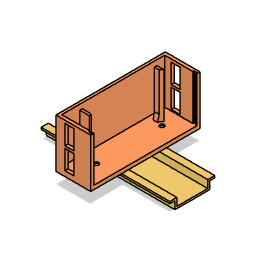
WLEDBoardMount (Autodesk Fusion 360 design; units mm, degrees)
Autodesk Fusion 360 part; units mm, degrees
sketch "Skizze1" plane through (0, 0, 0) normal (1, 0, 0) x (0, 0, -1) in component "Rail"
  line L0 (-17.5, 0) -> (17.5, 0)
  line L1 (-12, 0) -> (-12, -6)
  line L2 (-12, -6) -> (12, -6)
  line L3 (13.5, -1.5) -> (17.5, -1.5)
  line L4 (17.5, 0) -> (17.5, -1.5)
  line L5 (12, -6) -> (12, 0)
  line L6 (13.5, -7.5) -> (13.5, -1.5)
  line L7 (0, -7.5) -> (0, 0) construction
  line L8 (-17.5, 0) -> (-17.5, -1.5)
  line L9 (-17.5, -1.5) -> (-13.5, -1.5)
  line L10 (-13.5, -1.5) -> (-13.5, -7.5)
  line L11 (-13.5, -7.5) -> (13.5, -7.5)
  point P0 (0, -26.5)
  point P1 (5, -20.5)
  point P2 (5, -17.5)
  point P3 (-5, -17.5)
  point P4 (5, -20.5)
  point P5 (5, -17.5)
  point P6 (0, -26.5)
  point P7 (0, -8.5)
  point P8 (0, -14.5)
  point P9 (0, -35.0071)
  point P10 (0, -2.5)
  point P11 (0, 3.5)
  point P12 (0, 27.7571)
  point P13 (0, -0.2)
  point P14 (0, -8.5)
  point P15 (0, -14.5)
  point P16 (0, -35.0071)
  point P17 (0, -2.5)
  point P18 (0, 3.5)
  point P19 (0, 27.7571)
  point P20 (0, -0.2)
  point P21 (0, 24.5)
  point P22 (0, 24.5)
  point P23 (-50, 12)
  point P24 (50, 12)
  point P25 (50, 17.5)
  point P26 (-50, 17.5)
  point P27 (0, -24.5)
  point P28 (0, 26.5)
  point P29 (0, -26.5)
  point P30 (0, 24.5)
  point P31 (-7.5, 4)
  point P32 (-7.5, 39)
  dimension "d58" = 1
  dimension "d59" = 5
  constraint horizontal L0
  constraint midpoint L7.end L0
  constraint horizontal L11
  constraint midpoint L7.start L11
  constraint coincident L7.end origin
  constraint vertical L7
  constraint perpendicular L0 L8
  constraint perpendicular L0 L4
  constraint perpendicular L6 L11
  constraint perpendicular L3 L4
  constraint perpendicular L6 L9
  constraint perpendicular L9 L10
  constraint equal L4 L8
  constraint coincident L1.start L0
  constraint perpendicular L0 L1
  constraint perpendicular L2 L6
  constraint coincident L5.end L0
  constraint perpendicular L0 L5
  measures "d1" distance of L0.start L0.end
  measures "d2" distance of L10.end L6.start
  measures "d3" distance of L3.end L0.end
  measures "d4" distance of L0 L11
  measures "d5" distance of L2 L11
  measures "d6" distance of L1 L10
  measures "d7" distance of L5 L6
extrude "Extrusion1" add sketch "Skizze1" along normal mid plane 100 contours L0 L1 L2 L3 L4 L5 L6 L8 L9 L10 L11 makes body 1 in component "Rail"
sketch "Skizze1 (2)" plane through (0, 0, 0) normal (0, 1, 0) x (1, 0, 0) in component "DinRailMount"
  line L0 (-80, 17.5) -> (80, 17.5)
  line L1 (-80, 12) -> (80, 12)
  line L2 (-80, -12) -> (80, -12)
  line L3 (80, -17.5) -> (-80, -17.5)
  line L4 (0, 17.5) -> (0, -17.5) construction
  line L5 (-5, 17.5) -> (5, 17.5)
  line L6 (5, 17.5) -> (5, 20.5)
  line L7 (5, 20.5) -> (-5, 20.5)
  line L8 (-5, 20.5) -> (-5, 17.5)
  arc A0 (0, 17.5) -> (0, 11.5) centre (0, 14.5) ccw
  arc A1 (0, 5.5) -> (0, 11.5) centre (0, 8.5) ccw
  arc A2 (0, 5.5) -> (0, -0.5) centre (0, 2.5) ccw
  arc A3 (0, -6.5) -> (0, -0.5) centre (0, -3.5) ccw
  arc A4 (0, -5.8) -> (0, -1.2) centre (0, -3.5) ccw
  arc A5 (0, 6.2) -> (0, -1.2) centre (0, 2.5) ccw
  arc A6 (0, 6.2) -> (0, 10.8) centre (0, 8.5) ccw
  arc A7 (0, 18.2) -> (0, 10.8) centre (0, 14.5) ccw
  arc A8 (0, 16.8) -> (0, 12.2) centre (0, 14.5) ccw
  arc A9 (0, 4.8) -> (0, 12.2) centre (0, 8.5) ccw
  arc A10 (0, 4.8) -> (0, 0.2) centre (0, 2.5) ccw
  arc A11 (0, -7.2) -> (0, 0.2) centre (0, -3.5) ccw
  arc A12 (0, 16.8) -> (5, 17.5) centre (0, 35.0071) ccw
  line L9 (-8.5, 22.5) -> (8.5, 22.5) construction
  line L10 (8.5, 22.5) -> (8.5, -20.5)
  line L11 (8.5, -20.5) -> (-8.5, -20.5) construction
  line L12 (-8.5, -20.5) -> (-8.5, 22.5)
  line L13 (0, -17.5) -> (0, -20.5) construction
  line L14 (-5.5, 22.5) -> (5.5, 22.5)
  line L15 (5.5, 22.5) -> (5.5, -6.5)
  line L16 (5.5, -6.5) -> (-5.5, -6.5)
  line L17 (-5.5, -6.5) -> (-5.5, 22.5)
  arc A13 (0, -5.8) -> (-5.5, -6.5) centre (0, -27.7571) ccw
  line L18 (8.5, 22.5) -> (8.5, 30.5)
  line L19 (8.5, 30.5) -> (-8.5, 30.5)
  line L20 (-8.5, 30.5) -> (-8.5, 22.5)
  line L21 (0, 30.5) -> (0, 22.5) construction
  circle A14 centre (0, 26.5) radius 1.75
  line L22 (-8.5, -20.5) -> (-8.5, -28.5)
  line L23 (-8.5, -28.5) -> (8.5, -28.5)
  line L24 (8.5, -28.5) -> (8.5, -20.5)
  circle A15 centre (0, -24.5) radius 1.75
  line L25 (0, -28.5) -> (0, -20.5) construction
  line L26 (-50, 12) -> (50, 12)
  line L27 (50, 12) -> (50, 17.5)
  line L28 (50, 17.5) -> (-50, 17.5)
  line L29 (-50, 17.5) -> (-50, 12)
  dimension "d89_1" = 10
  dimension "d91_1" = 3
  dimension "d94_1" = 3
  dimension "d95_1" = 6
  dimension "d98_1" = 0
  dimension "d99_1" = -12
  dimension "d100_1" = 0.7
  dimension "d101_1" = -0.7
  dimension "d102_1" = 5
  dimension "d103_1" = 3
  dimension "d105_1" = 2
  dimension "d106_1" = 3.5
  dimension "d107_1" = 4
  dimension "d111_1" = 0.5
  dimension "d149_1" = 3
  constraint midpoint L0 L4.start
  constraint midpoint L3 L4.end
  constraint horizontal L5
  constraint vertical L6
  constraint horizontal L7
  constraint vertical L8
  constraint coincident L0 L5.start
  constraint midpoint L4.start L5
  constraint coincident L4 A0.end
  constraint coincident L4 A0.centre
  constraint coincident L4 A1.start
  constraint coincident L4 A1.centre
  constraint tangent A8 A12
  constraint horizontal L9
  constraint vertical L10
  constraint horizontal L11
  constraint vertical L12
  constraint midpoint L11 L13.end
  constraint collinear L4 L13
  constraint horizontal L14
  constraint vertical L15
  constraint horizontal L16
  constraint vertical L17
  constraint midpoint A3.start L16
  constraint tangent A4 A13
  constraint vertical L18
  constraint horizontal L19
  constraint vertical L20
  constraint coincident L9.end L10.start
  constraint midpoint L19 L21.start
  constraint midpoint L21 A14.centre
  constraint midpoint L14 L21.end
  constraint perpendicular L11 L22
  constraint perpendicular L22 L23
  constraint perpendicular L23 L24
  constraint equal L20 L22
  constraint equal A14 A15
  constraint midpoint L23 L25.start
  constraint midpoint A15.centre L25
  measures "d89_1" distance of L5.start L5.end
  measures "d91_1" distance of L5.end L6.end
  measures "d94_1" distance of L5 A0.centre
  measures "d95_1" distance of A0.centre A1.centre
  measures "d102_1" distance of L0 L9
  measures "d103_1" distance of L3 L11
  measures "d105_1" distance of L7 L14
  measures "d106_1" diameter of A14
  measures "d107_1" distance of L19 A14.centre
  measures "d111_1" distance of L8 L17
  measures "d149_1" distance of L12 L17
extrude "Extrusion1'" add sketch "Skizze1 (2)" along normal blind 3 separate body contours L0 L5 L6 L7 L8 L28 | L0 L1 L5 A0 A7 L26 L28 | L0 L1 L5 A0 A8 A9 A12 L26 L28 | L1 A0 A1 A2 A3 A4 A5 A6 A7 L16 A13 L26 | L1 A0 A1 A2 A3 A9 A10 A11 L16 L26 | L0 L10 L12 L14 L15 L17 L18 L19 L20 L28 | L0 L1 L10 L15 L26 L28 | L1 L2 L10 L12 L15 L16 L17 L26 | L0 L1 L12 L17 L26 L28 | L2 L3 L10 L12 | L3 L10 L12 L22 L23 L24 makes body 2 in component "DinRailMount"
sketch "Skizze2" plane through (0, 3, 0) normal (0, 1, 0) x (-1, 0, 0) in component "DinRailMount"
  circle A0 centre (0, -26.5) radius 1.75
  line L0 (5.5, 6.5) -> (5.5, -22.5)
  line L1 (5.5, -22.5) -> (-5.5, -22.5)
  line L2 (-5.5, -22.5) -> (-5.5, 6.5)
  line L3 (-5.5, 6.5) -> (-2.1656, 6.5)
  line L4 (-8.5, 28.5) -> (-8.5, -30.5)
  line L5 (-8.5, -30.5) -> (8.5, -30.5)
  line L6 (8.5, -30.5) -> (8.5, 28.5)
  line L7 (5, -17.5) -> (6, -17.5)
  line L8 (6, -17.5) -> (6, -22)
  line L9 (6, -22) -> (5.5, -22)
  line L10 (5, -20.5) -> (6, -20.5)
  line L11 (5, -17) -> (6.5, -17)
  line L12 (6.5, -17) -> (6.5, -22.5)
  line L13 (6.5, -22.5) -> (5.5, -22.5)
  line L14 (-5, -17.5) -> (-6, -17.5)
  line L15 (-6, -17.5) -> (-6, -22)
  line L16 (-6, -22) -> (-5.5, -22)
  line L17 (-5, -20.5) -> (-6, -20.5)
  line L18 (-5, -17) -> (-6.5, -17)
  line L19 (-6.5, -17) -> (-6.5, -22.5)
  line L20 (-6.5, -22.5) -> (-5.5, -22.5)
  line L21 (5, -20.5) -> (5, -17.5)
  line L22 (5, -17.5) -> (2.1656, -17.5)
  line L23 (-5, -17.5) -> (-5, -20.5)
  line L24 (-5, -20.5) -> (5, -20.5)
  line L25 (-5, -17.5) -> (-5, -20.5)
  line L26 (-5, -20.5) -> (5, -20.5)
  line L27 (5, -20.5) -> (5, -17.5)
  line L28 (5, -17.5) -> (2.1656, -17.5)
  line L29 (-8.5, 28.5) -> (-8.5, -30.5)
  line L30 (-8.5, -30.5) -> (8.5, -30.5)
  line L31 (8.5, -30.5) -> (8.5, 28.5)
  circle A1 centre (0, -26.5) radius 1.75
  line L32 (5.5, 6.5) -> (5.5, -22.5)
  line L33 (5.5, -22.5) -> (-5.5, -22.5)
  line L34 (-5.5, -22.5) -> (-5.5, 6.5)
  line L35 (-5.5, 6.5) -> (-2.1656, 6.5)
  arc A2 (0, -4.8) -> (0, -12.2) centre (0, -8.5) ccw
  arc A3 (0, -16.8) -> (0, -12.2) centre (0, -14.5) ccw
  arc A4 (0, -16.8) -> (-5, -17.5) centre (0, -35.0071) ccw
  arc A5 (2.1656, -17.5) -> (0, -10.8) centre (0, -14.5) ccw
  arc A6 (0, -6.2) -> (0, -10.8) centre (0, -8.5) ccw
  arc A7 (0, -6.2) -> (0, 1.2) centre (0, -2.5) ccw
  arc A8 (0, 5.8) -> (0, 1.2) centre (0, 3.5) ccw
  arc A9 (0, 5.8) -> (5.5, 6.5) centre (0, 27.7571) ccw
  arc A10 (-2.1656, 6.5) -> (0, -0.2) centre (0, 3.5) ccw
  arc A11 (0, -4.8) -> (0, -0.2) centre (0, -2.5) ccw
  arc A12 (0, -4.8) -> (0, -12.2) centre (0, -8.5) ccw
  arc A13 (0, -16.8) -> (0, -12.2) centre (0, -14.5) ccw
  arc A14 (0, -16.8) -> (-5, -17.5) centre (0, -35.0071) ccw
  arc A15 (2.1656, -17.5) -> (0, -10.8) centre (0, -14.5) ccw
  arc A16 (0, -6.2) -> (0, -10.8) centre (0, -8.5) ccw
  arc A17 (0, -6.2) -> (0, 1.2) centre (0, -2.5) ccw
  arc A18 (0, 5.8) -> (0, 1.2) centre (0, 3.5) ccw
  arc A19 (0, 5.8) -> (5.5, 6.5) centre (0, 27.7571) ccw
  arc A20 (-2.1656, 6.5) -> (0, -0.2) centre (0, 3.5) ccw
  arc A21 (0, -4.8) -> (0, -0.2) centre (0, -2.5) ccw
  line L36 (8.5, 28.5) -> (-8.5, 28.5)
  line L37 (8.5, 28.5) -> (-8.5, 28.5)
  circle A22 centre (0, 24.5) radius 1.75
  circle A23 centre (0, 24.5) radius 1.75
  dimension "d119_1" = 0.5
  dimension "d120_1" = -0.5
  dimension "d121_1" = 0.5
  dimension "d148_1" = 0.5
  constraint perpendicular L1 L8
  constraint perpendicular L0 L9
  constraint coincident L8 L10.end
  constraint perpendicular L8 L10
  constraint coincident L0 L9.end
  constraint coincident L1 L0.end
  constraint perpendicular L2 L14
  constraint perpendicular L14 L15
  constraint coincident L2 L16.end
  constraint perpendicular L2 L16
  constraint coincident L15 L17.end
  constraint perpendicular L15 L17
  constraint equal L7 L14
  constraint equal L8 L15
  measures "d119_1" distance of L0 L8
  measures "d121_1" distance of L1 L9
extrude "Extrusion2" cut sketch "Skizze2" against normal blind 1.4 from surface at -0.5 contours L0 L7 L8 L9 L11 L12 L13 L32 | L0 L8 L9 L10 L32 | L0 L7 L8 L10 L32 | L2 L14 L15 L16 L18 L19 L20 L34 | L2 L15 L16 L17 L34 | L2 L14 L15 L17 L34 bodies 2 in component "DinRailMount"
extrude "Extrusion3" add sketch "Skizze2" along normal blind 1 from surface at -1.7 contours L0 L7 L10 L21 L27 L32 | L0 L7 L8 L10 L32 | L2 L14 L17 L23 L25 L34 | L2 L14 L15 L17 L34 bodies 2 in component "DinRailMount"
sketch "Skizze3" plane through (5, 0, 0) normal (1, 0, 0) x (0, 0, -1) in component "DinRailMount"
  line L0 (20.5, 1.3) -> (17.5, 1.3)
  line L1 (17.5, 0) -> (20.5, 0)
  line L2 (20.5, 0) -> (20.5, 1.3)
  line L3 (20.5, 0) -> (20.5, -2)
  line L4 (16, -2) -> (16, -1.5)
  line L5 (16, -2) -> (17, -3)
  line L6 (17, -3) -> (19.5, -3)
  line L7 (19.5, -3) -> (20.5, -2)
  line L8 (20.5, -2) -> (16, -2) construction
  line L9 (17.5, 1.3) -> (17.5, 0)
  line L10 (-17.5, 0) -> (-17.5, -1.5)
  line L11 (-17.5, -1.5) -> (-13.5, -1.5)
  line L12 (-13.5, -1.5) -> (-13.5, -7.5)
  line L13 (-13.5, -7.5) -> (13.5, -7.5)
  line L14 (13.5, -7.5) -> (13.5, -1.5)
  line L15 (13.5, -1.5) -> (17.5, -1.5)
  line L16 (17.5, -1.5) -> (17.5, 0)
  line L17 (17.5, 0) -> (12, 0)
  line L18 (12, 0) -> (12, -6)
  line L19 (12, -6) -> (-12, -6)
  line L20 (-12, -6) -> (-12, 0)
  line L21 (-12, 0) -> (-17.5, 0)
  dimension "d127_1" = 1.5
  dimension "d129_1" = 0.5
  dimension "d130_1" = 1.5
  dimension "d151_1" = 45
  dimension "d152_1" = 45
  constraint coincident L1.end L2.start
  constraint perpendicular L1 L3
  constraint coincident L4.end L15
  constraint perpendicular L4 L15
  constraint horizontal L6
  constraint perpendicular L4 L8
  measures "d127_1" distance of L4 L16
  measures "d129_1" distance of L4.start L4.end
  measures "d130_1" distance of L6 L15
  measures "d151_1" angle of L5 L8
  measures "d152_1" angle of L7 L8
extrude "Extrusion4" add sketch "Skizze3" against normal up to surface (10 mm away) contours L1 L3 L4 L5 L6 L7 L15 L16 bodies 2 in component "DinRailMount"
sketch "Skizze4" plane through (8.5, 0, 0) normal (1, 0, 0) x (0, 0, -1) in component "DinRailMount"
  line L0 (-28.5, 0) -> (30.5, 0)
  line L1 (30.5, 0) -> (30.5, 3)
  line L2 (30.5, 3) -> (-28.5, 3)
  line L3 (-20, -3) -> (-21, -2)
  line L4 (-17, -3) -> (-20, -3)
  line L5 (-16, -2) -> (-17, -3)
  line L6 (-16, -2) -> (-16, -1.5)
  line L7 (-16, -2) -> (-21, -2) construction
  line L8 (-28.5, 3) -> (-28.5, 0)
  line L9 (-21, -2) -> (-21, 0)
  line L10 (-17.5, 0) -> (-17.5, -1.5)
  line L11 (-17.5, -1.5) -> (-13.5, -1.5)
  line L12 (-13.5, -1.5) -> (-13.5, -7.5)
  line L13 (-13.5, -7.5) -> (13.5, -7.5)
  line L14 (13.5, -7.5) -> (13.5, -1.5)
  line L15 (13.5, -1.5) -> (17.5, -1.5)
  line L16 (17.5, -1.5) -> (17.5, 0)
  line L17 (17.5, 0) -> (12, 0)
  line L18 (12, 0) -> (12, -6)
  line L19 (12, -6) -> (-12, -6)
  line L20 (-12, -6) -> (-12, 0)
  line L21 (-12, 0) -> (-17.5, 0)
  dimension "d141_1" = 0.5
  dimension "d143_1" = 1.5
  dimension "d144_1" = 1.5
  dimension "d153_1" = 45
  dimension "d154_1" = 45
  dimension "d238_1" = 5
  constraint coincident L6.end L11
  constraint perpendicular L6 L11
  constraint perpendicular L6 L7
  constraint coincident L0 L9.end
  constraint perpendicular L0 L9
  measures "d141_1" distance of L5.start L6.end
  measures "d143_1" distance of L4 L11
  measures "d144_1" distance of L6 L10
  measures "d153_1" angle of L3 L7
  measures "d154_1" angle of L5 L7
  measures "d238_1" distance of L6 L9
extrude "Extrusion5" add sketch "Skizze4" against normal up to surface (17 mm away) contours L0 L3 L4 L5 L6 L9 L10 L11 bodies 2 in component "DinRailMount"
ref_plane "Arbeitsebene1" through (0, 1, -1) normal (0, 1, 0) x (1, 0, 0) in component "DinRailMount"
sketch "Skizze1 (3)" plane through (0, 1, 0) normal (0, 1, 0) x (1, 0, 0) in component "MainBody"
  line L0 (-13.5, 42.5) -> (13.5, 42.5)
  line L1 (13.5, 42.5) -> (13.5, -42.5)
  line L2 (13.5, -42.5) -> (-13.5, -42.5)
  line L3 (-13.5, -42.5) -> (-13.5, 42.5)
  line L4 (-13.5, 42.5) -> (13.5, -42.5) construction
  line L5 (13.5, 42.5) -> (-13.5, -42.5) construction
  line L6 (8.5, -28.5) -> (8.5, 30.5)
  line L7 (-8.5, -28.5) -> (8.5, -28.5)
  circle A0 centre (0, -24.5) radius 1.75
  line L8 (-8.5, 30.5) -> (-8.5, -28.5)
  line L9 (8.5, 30.5) -> (-8.5, 30.5)
  circle A1 centre (0, 26.5) radius 1.75
  dimension "d10" = 27
  dimension "d11" = 85
  constraint horizontal L0
  constraint perpendicular L0 L1
  constraint parallel L0 L2
  constraint parallel L1 L3
  constraint coincident L4 origin
  constraint coincident L5 origin
  measures "d10" distance of L1.end L2.end
  measures "d11" distance of L0.end L1.end
extrude "Extrusion1''" add sketch "Skizze1 (3)" along normal blind 3 separate body contours L0 L1 L2 L3 | L6 L7 L8 L9 makes body 3 in component "MainBody"
extrude "Extrusion2'" cut sketch "Skizze1 (3)" along normal up to surface (2 mm away) contours L6 L7 L8 L9 bodies 3 in component "MainBody"
sketch "Skizze2 (2)" plane through (0, 4, 0) normal (0, 1, 0) x (-1, 0, 0) in component "MainBody"
  circle A0 centre (0, -26.5) radius 1.75
  circle A1 centre (0, 24.5) radius 1.75
  line L0 (13.5, 42.5) -> (-13.5, 42.5)
  line L1 (-13.5, 42.5) -> (-13.5, -42.5)
  line L2 (-13.5, -42.5) -> (13.5, -42.5)
  line L3 (13.5, -42.5) -> (13.5, 42.5)
  line L4 (-11.5, -40) -> (11.5, -40)
  line L5 (11.5, -40) -> (11.5, 40)
  line L6 (11.5, 40) -> (-11.5, 40)
  line L7 (-11.5, 40) -> (-11.5, -40) construction
  line L8 (-11.5, -40) -> (11.5, 40) construction
  line L9 (11.5, -40) -> (-11.5, 40) construction
  line L10 (7.5, -30) -> (7.5, -28)
  line L11 (1.9365, -30) -> (7.5, -30)
  line L12 (7.5, -28) -> (3.7081, -28)
  arc A2 (1.9365, -30) -> (3.7081, -28) centre (0, -26.5) ccw
  line L13 (7.5, 28) -> (1.9365, 28)
  line L14 (0, 28.5) -> (0, 30)
  line L15 (0, 30) -> (7.5, 30)
  line L16 (7.5, 30) -> (7.5, 28)
  line L17 (0, 24.5) -> (0, 28.5) construction
  arc A3 (1.9365, 28) -> (0, 28.5) centre (0, 24.5) ccw
  line L18 (-12.5, -41) -> (-10.5, -41)
  line L19 (-10.5, -41) -> (-10.5, -40)
  line L20 (-12.5, -41) -> (-12.5, -40)
  line L21 (-10.5, 40) -> (-10.5, 41)
  line L22 (-10.5, 41) -> (-12.5, 41)
  line L23 (-12.5, 41) -> (-12.5, 40)
  line L24 (-11.5, -40) -> (-13.5, -40)
  line L25 (-11.5, 40) -> (-13.5, 40)
  dimension "d18" = 2
  dimension "d19" = 80
  dimension "d31" = 8
  dimension "d32" = 2
  dimension "d33" = 10
  dimension "d35" = 10
  dimension "d62" = 1.5
  dimension "d64" = 2
  dimension "d65" = 1
  dimension "d66" = 4
  constraint horizontal L4
  constraint perpendicular L4 L5
  constraint parallel L4 L6
  constraint parallel L5 L7
  constraint coincident L8 origin
  constraint coincident L9 origin
  constraint vertical L10
  constraint horizontal L12
  constraint coincident A0.centre A2.centre
  constraint horizontal L11
  constraint horizontal L13
  constraint vertical L14
  constraint horizontal L15
  constraint vertical L16
  constraint concentric A1 A3
  constraint collinear L10 L16
  constraint equal L10 L16
  constraint coincident A1.centre L17.start
  constraint vertical L17
  constraint coincident L14.start L17.end
  constraint equal A2 A3
  constraint coincident L4 L20.end
  constraint perpendicular L4 L20
  constraint perpendicular L21 L22
  constraint coincident L6 L23.end
  constraint perpendicular L6 L23
  constraint collinear L19 L21
  constraint equal L18 L22
  constraint equal L20 L23
  constraint coincident L1 L24.end
  constraint perpendicular L1 L24
  constraint coincident L1 L25.end
  constraint perpendicular L1 L25
  constraint coincident L12.end A2.end
  constraint coincident L11.start A2.start
  constraint coincident L13.end A3.start
  constraint coincident L6 L21.start
  constraint coincident L4 L19.end
  measures "d18" distance of L1 L7
  measures "d19" distance of L4.start L6.end
  measures "d31" diameter of A2
  measures "d32" distance of L11 L12
  measures "d33" distance of L4 L11
  measures "d35" distance of L6 L15
  measures "d62" distance of L2 L18
  measures "d64" distance of L18.start L18.end
  measures "d65" distance of L1 L20
  measures "d66" distance of L5 L10
extrude "Extrusion3'" add sketch "Skizze2 (2)" along normal blind 35 contours L0 L1 L2 L3 L4 L5 L6 L18 L19 L20 L21 L22 L23 L24 L25 | L10 L11 L12 A2 | L13 L14 L15 L16 A3 bodies 3 in component "MainBody"
chamfer "Fase1" distance 1 distance2 5 2 edges at (-5.604, 4, -28) (-4.7182, 4, 28) measured on face at (9.5256, 4, 7.9136) measured on face at (9.5256, 4, 7.9136) on bodies 3 in component "MainBody"
sketch "Skizze5" plane through (0, 0, -42.5) normal (0, 0, -1) x (-1, 0, 0) in component "MainBody"
  line L0 (-13.5, 1) -> (13.5, 1)
  line L1 (13.5, 1) -> (13.5, 39)
  line L2 (13.5, 39) -> (-13.5, 39)
  line L3 (-13.5, 39) -> (-13.5, 1)
  line L4 (-0.5, 20) -> (6.5, 20)
  line L5 (6.5, 20) -> (6.5, 5)
  line L6 (6.5, 5) -> (-0.5, 5)
  line L7 (-0.5, 5) -> (-0.5, 20)
  line L8 (7.5, 4) -> (7.5, 39)
  line L9 (-0.5, 36.8) -> (6.5, 36.8)
  line L10 (6.5, 36.8) -> (6.5, 21.8)
  line L11 (6.5, 21.8) -> (-0.5, 21.8)
  line L12 (-0.5, 21.8) -> (-0.5, 36.8)
  line L13 (-10.5, 4) -> (11.5, 4)
  line L14 (11.5, 4) -> (11.5, 39)
  dimension "d45" = 1.8
  dimension "d46" = 7
  dimension "d47" = 15
  dimension "d67" = 1
  dimension "d68" = 1
  constraint horizontal L4
  constraint vertical L5
  constraint horizontal L6
  constraint vertical L7
  constraint horizontal L9
  constraint vertical L10
  constraint horizontal L11
  constraint vertical L12
  constraint equal L5 L10
  constraint equal L4 L9
  constraint collinear L7 L12
  measures "d45" distance of L4 L11
  measures "d46" distance of L9.start L9.end
  measures "d47" distance of L9.end L10.end
  measures "d67" distance of L5 L8
  measures "d68" distance of L6 L13
extrude "Extrusion5'" cut sketch "Skizze5" against normal up to surface (2.5 mm away) contours L4 L5 L6 L7 | L9 L10 L11 L12 bodies 3 in component "MainBody"
sketch "Skizze6" plane through (0, 0, 42.5) normal (0, 0, 1) x (1, 0, 0) in component "MainBody"
  line L0 (-13.5, 1) -> (13.5, 1)
  line L1 (13.5, 1) -> (13.5, 39)
  line L2 (13.5, 39) -> (-13.5, 39)
  line L3 (-13.5, 39) -> (-13.5, 1)
  line L4 (-6.5, 20) -> (0.5, 20)
  line L5 (0.5, 20) -> (0.5, 5)
  line L6 (0.5, 5) -> (-6.5, 5)
  line L7 (-6.5, 5) -> (-6.5, 20)
  line L8 (-6.5, 36.8) -> (0.5, 36.8)
  line L9 (0.5, 36.8) -> (0.5, 21.8)
  line L10 (0.5, 21.8) -> (-6.5, 21.8)
  line L11 (-6.5, 21.8) -> (-6.5, 36.8)
  line L12 (-7.5, 4) -> (-7.5, 39)
  line L13 (-11.5, 4) -> (10.5, 4)
  line L14 (-11.5, 4) -> (-11.5, 39)
  dimension "d51" = 7
  dimension "d52" = 15
  dimension "d55" = 1.8
  dimension "d69" = 1
  dimension "d70" = 1
  constraint horizontal L4
  constraint vertical L5
  constraint horizontal L6
  constraint vertical L7
  constraint horizontal L8
  constraint vertical L9
  constraint horizontal L10
  constraint vertical L11
  constraint collinear L5 L9
  constraint equal L7 L11
  constraint equal L4 L8
  measures "d51" distance of L8.start L8.end
  measures "d52" distance of L8.start L10.end
  measures "d55" distance of L4 L10
  measures "d69" distance of L6 L13
  measures "d70" distance of L7 L12
extrude "Extrusion6" cut sketch "Skizze6" against normal up to surface (2.5 mm away) contours L4 L5 L6 L7 | L8 L9 L10 L11 bodies 3 in component "MainBody"
component "Rail" placed x (1, 0, 0) y (0, 1, 0) z (0, 0, 1) at (0, 0, 0)
component "DinRailMount" placed x (1, 0, 0) y (0, 1, 0) z (0, 0, 1) at (0, 0, 0)
component "MainBody" placed x (1, 0, 0) y (0, 1, 0) z (0, 0, 1) at (0, 0, 0)
